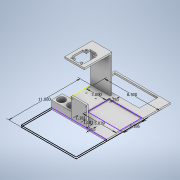
# Autodesk Inventor part: liquid cell loader tray thing
Saved by Autodesk Inventor 2020 (Build 240168000, 168)
## iProperties
Created: 2021-12-08
Part Number: liquid cell loader tray thing
Material: Generic
Document SubType Name: Modeling
Designer: pab2
Density: 1 g/cm^3
Appearance: Default
Author: pab2
Autodesk Inventor part; units mm, degrees
ref_plane "YZ Plane" through (0, 0, 0) normal (1, 0, 0) x (0, 1, 0)
ref_plane "XZ Plane" through (0, 0, 0) normal (0, 1, 0) x (-1, 0, 0)
ref_plane "XY Plane" through (0, 0, 0) normal (0, 0, 1) x (1, 0, 0)
sketch "Sketch1" plane through (0, 0, 0) normal (0, 1, 0) x (-1, 0, 0)
  line L0 (0, 0) -> (215.9, 0)
  line L1 (215.9, 0) -> (215.9, -279.4)
  line L2 (215.9, -279.4) -> (0, -279.4)
  line L3 (0, -279.4) -> (0, 0)
  line L4 (215.9, -279.4) -> (139.7, -279.4)
  line L5 (139.7, -279.4) -> (139.7, -273.05)
  line L6 (139.7, -273.05) -> (215.9, -273.05)
  line L7 (215.9, -273.05) -> (215.9, -279.4)
  dimension "d0" = 215.9
  dimension "d1" = 279.4
  dimension "d2" = 76.2
  dimension "d3" = 6.35
  constraints: 16 end point, 4 parallel, 2 horizontal, 2 perpendicular
  measures "d0" distance of L1.end L2.end
  measures "d1" distance of L0.end L1.end
  measures "d2" distance of L5.end L6.end
  measures "d3" distance of L4.end L5.end
extrude "Extrusion1" add sketch "Sketch1" along normal blind 152.4 contours L1 L2 L5 L6
extrude "Extrusion2" add sketch "Sketch1" along normal blind 6.35 contours L0 L1 L6 L5 L2 L3
sketch "Sketch2" plane through (-215.9, 152.4, -273.05) normal (0, 0, 1) x (1, 0, 0)
  line L0 (76.2, 0) -> (0, 0) projected
  line L1 (76.2, -146.05) -> (76.2, 0) projected
  line L2 (0, 0) -> (76.2, 0)
  line L3 (76.2, 0) -> (76.2, -6.35)
  line L4 (76.2, -6.35) -> (0, -6.35)
  line L5 (0, -6.35) -> (0, 0)
  point P0 (215.9, -152.4)
  dimension "d8" = 6.35
  constraints: 8 end point, 2 parallel, 1 horizontal, 1 perpendicular, 1 point on line
  measures "d8" distance of L2.end L3.end
extrude "Extrusion3" add sketch "Sketch2" along normal blind 101.6
sketch "Sketch3" plane through (0, 152.4, 0) normal (0, 1, 0) x (1, 0, 0)
  line L0 (-215.9, 273.05) -> (-215.9, 0) projected
  line L1 (-139.7, 171.45) -> (-215.9, 171.45)
  line L2 (-215.9, 171.45) -> (-215.9, 180.975)
  line L3 (-215.9, 180.975) -> (-139.7, 180.975)
  line L4 (-139.7, 180.975) -> (-139.7, 171.45)
  line L5 (-177.8, 180.975) -> (-196.088, 180.975)
  line L6 (-177.8, 180.975) -> (-159.512, 180.975)
  line L7 (-159.512, 180.975) -> (-159.512, 236.601)
  line L8 (-196.088, 180.975) -> (-196.088, 236.601)
  point P0 (0, 0)
  dimension "d11" = 9.525
  dimension "d12" = 18.288
  dimension "d13" = 18.288
  dimension "d14" = 55.626
  dimension "d15" = 55.626
  constraints: 16 end point, 3 point on line, 2 parallel, 2 perpendicular, 1 horizontal, 1 midpoint, 1 vertical
  measures "d11" distance of L1.end L2.end
  measures "d12" distance of L5.start L5.end
  measures "d13" distance of L5.start L6.end
  measures "d14" distance of L6.end L7.end
  measures "d15" distance of L5.end L8.end
hole "Hole1" at (-196.088, 152.4, -236.601) at (-159.512, 152.4, -236.601) at (-159.512, 152.4, -180.975) at (-196.088, 152.4, -180.975) direction (0, -1, 0) diameter 4.4958 depth 146.05 tip angle 118 start extended yes counterbore diameter 7.9502 counterbore depth 4.1656 clearance for "Socket Head Cap Screw" size "#8" standard "Ansi Unified Screw Threads"
sketch "Sketch4" plane through (0, 152.4, 0) normal (0, 1, 0) x (1, 0, 0)
  line L0 (-215.9, 279.4) -> (-215.9, 171.45) projected
  line L1 (-215.9, 171.45) -> (-215.9, 187.325)
  line L2 (-215.9, 187.325) -> (-203.2, 187.325)
  line L3 (-203.2, 187.325) -> (-153.924, 187.325)
  line L4 (-153.924, 187.325) -> (-153.924, 229.8268)
  line L5 (-153.924, 229.8268) -> (-203.2, 229.8268)
  line L6 (-203.2, 229.8268) -> (-203.2, 187.325)
  line L7 (-190.2248, 177.0242) -> (-165.5159, 177.0242)
  line L8 (-165.5159, 177.0242) -> (-165.5159, 245.3968)
  line L9 (-165.5159, 245.3968) -> (-190.2248, 245.3968)
  line L10 (-190.2248, 245.3968) -> (-190.2248, 177.0242)
  point P0 (0, 0)
  point P1 (-165.5159, 187.325)
  point P2 (-165.5159, 229.8268)
  point P3 (-190.2248, 229.8268)
  point P4 (-190.2248, 187.325)
  dimension "d23" = 15.875
  dimension "d24" = 12.7
  dimension "d25" = 49.276
  constraints: 20 end point, 4 parallel, 3 perpendicular, 2 horizontal, 1 point on line
  measures "d23" distance of L0.end L1.end
  measures "d24" distance of L1.end L2.end
  measures "d25" distance of L5.end L4.end
extrude "Extrusion4" cut sketch "Sketch4" against normal blind 101.6
sketch "Sketch5" plane through (0, 6.35, 0) normal (0, 1, 0) x (1, 0, 0)
  line L0 (-132.2495, 261.4471) -> (-4.2495, 261.4471)
  line L1 (-4.2495, 261.4471) -> (-4.2495, 175.4471)
  line L2 (-4.2495, 175.4471) -> (-132.2495, 175.4471)
  line L3 (-132.2495, 175.4471) -> (-132.2495, 261.4471)
  line L4 (-215.9, 273.05) -> (-215.9, 0) projected
  line L5 (-215.9, 161.7513) -> (-138.3533, 161.7513)
  line L6 (-138.3533, 161.7513) -> (-138.3533, 119.3637)
  line L7 (-138.3533, 119.3637) -> (-215.9, 119.3637)
  line L8 (-215.9, 119.3637) -> (-215.9, 161.7513)
  line L9 (-215.9, 119.3637) -> (0, 119.3637)
  line L10 (0, 119.3637) -> (0, 0)
  line L11 (0, 0) -> (-215.9, 0)
  line L12 (-215.9, 0) -> (-215.9, 119.3637)
  line L13 (-107.95, 119.3637) -> (-77.95, 119.3637)
  line L14 (-77.95, 119.3637) -> (-77.95, 125.7137)
  line L15 (-77.95, 125.7137) -> (-107.95, 125.7137)
  line L16 (-107.95, 125.7137) -> (-107.95, 119.3637)
  line L17 (-107.95, 119.3637) -> (-137.95, 119.3637)
  line L18 (-137.95, 119.3637) -> (-137.95, 125.7137)
  line L19 (-137.95, 125.7137) -> (-107.95, 125.7137)
  line L20 (-107.95, 125.7137) -> (-107.95, 119.3637)
  dimension "d28" = 128
  dimension "d29" = 86
  dimension "d42" = 30
  dimension "d43" = 6.35
  dimension "d44" = 30
  constraints: 40 end point, 10 parallel, 5 horizontal, 5 perpendicular, 1 midpoint, 1 point on line
  measures "d28" distance of L1.end L2.end
  measures "d29" distance of L0.end L1.end
  measures "d42" distance of L15.end L14.end
  measures "d43" distance of L14.end L13.end
  measures "d44" distance of L18.end L19.end
extrude "Extrusion5" cut sketch "Sketch5" against normal blind 3.81 contours L0 L1 L2 L3
extrude "Extrusion6" add sketch "Sketch5" along normal blind 25.4 contours L5 L6 L7 L4
sketch "Sketch6" plane through (0, 31.75, 0) normal (0, 1, 0) x (1, 0, 0)
  line L0 (-138.3533, 161.7513) -> (-138.3533, 119.3637) projected
  line L1 (-138.3533, 140.5575) -> (-157.4033, 140.5575)
  line L2 (-215.9, 279.4) -> (-215.9, 0) projected
  line L3 (-138.3533, 140.5575) -> (-119.3033, 140.5575) construction
  circle A0 centre (-157.4033, 140.5575) radius 14.5
  line L4 (-215.9, 139.7) -> (-196.85, 139.7)
  line L5 (-215.9, 139.7) -> (-196.85, 139.7) construction
  circle A1 centre (-196.85, 139.7) radius 14.5
  point P0 (0, 0)
  dimension "d34" = 19.05
  dimension "d35" = 180
  dimension "d36" = 29
  dimension "d37" = 19.05
  dimension "d38" = 0
  dimension "d39" = 29
  constraints: 8 end point, 3 horizontal, 2 centre point, 2 coincident, 2 collinear, 2 midpoint, 1 perpendicular
  measures "d34" distance of L1.start L1.end
  measures "d35" angle of L1 L3
  measures "d36" diameter of A0
  measures "d37" distance of L4.start L4.end
  measures "d38" distance between parallel lines of L4 L5
  measures "d39" diameter of A1
extrude "Extrusion7" cut sketch "Sketch6" against normal blind 29.21
extrude "Extrusion8" add sketch "Sketch5" along normal blind 76.2 contours L18 L19 L16 L9 | L16 L15 L14 L9
extrude "Extrusion9" cut sketch "Sketch5" against normal blind 76.2 contours L7 L9 L10 L11 L4
sketch "Sketch7" plane through (-215.9, 0, -119.3637) normal (0, 0, 1) x (1, 0, 0)
  line L0 (77.95, 82.55) -> (137.95, 82.55) projected
  line L1 (107.95, 82.55) -> (134.45, 82.55)
  line L2 (134.45, 82.55) -> (134.45, 76.2)
  line L3 (134.45, 76.2) -> (107.95, 76.2)
  line L4 (107.95, 76.2) -> (107.95, 82.55)
  line L5 (107.95, 82.55) -> (81.45, 82.55)
  line L6 (81.45, 82.55) -> (81.45, 76.2)
  line L7 (81.45, 76.2) -> (107.95, 76.2)
  line L8 (107.95, 76.2) -> (107.95, 82.55)
  point P0 (215.9, 0)
  point P1 (113.2316, 50.6759)
  point P2 (91.9547, 40.3217)
  dimension "d49" = 26.5
  dimension "d50" = 6.35
  dimension "d51" = 26.5
  constraints: 16 end point, 4 parallel, 2 horizontal, 2 perpendicular, 1 midpoint
  measures "d49" distance of L2.end L3.end
  measures "d50" distance of L1.end L2.end
  measures "d51" distance of L7.end L6.end
hole "Hole2" at (-134.45, 76.2, -119.3637) at (-81.45, 76.2, -119.3637) direction (0, 0, -1) diameter 3.683 depth 6.35 tip angle 118 start extended yes thread size "10-24 UNC" class "2B" standard "ANSI Unified Screw Threads"
sketch "Sketch9" plane through (-139.7, 152.4, -279.4) normal (0, 0, -1) x (-1, 0, 0)
  line L0 (-139.7, -146.05) -> (0, -146.05) projected
  line L1 (-139.7, -146.05) -> (76.2457, -146.05)
  line L2 (76.2457, -146.05) -> (76.2457, -152.4)
  line L3 (76.2457, -152.4) -> (-139.7, -152.4)
  line L4 (-139.7, -152.4) -> (-139.7, -146.05)
  constraints: 8 end point, 2 parallel, 1 horizontal, 1 perpendicular
extrude "Extrusion10" add sketch "Sketch9" along normal blind 88.9
sketch "Sketch10" plane through (0, 6.35, 0) normal (0, 1, 0) x (1, 0, 0)
  line L0 (-215.9457, 368.3) -> (0, 368.3) projected
  line L1 (-215.9457, 368.3) -> (-215.9457, 361.95)
  line L2 (-215.9457, 279.4) -> (-215.9457, 368.3) projected
  line L3 (-215.9457, 361.95) -> (-209.5957, 361.95)
  line L4 (-209.5957, 361.95) -> (-41.3207, 361.95)
  line L5 (-41.3207, 361.95) -> (-41.3207, 288.925)
  line L6 (-41.3207, 288.925) -> (-209.5957, 288.925)
  line L7 (-209.5957, 288.925) -> (-209.5957, 361.95)
  point P0 (0, 0)
  dimension "d61" = 6.35
  dimension "d62" = 6.35
  dimension "d63" = 168.275
  dimension "d64" = 73.025
  constraints: 12 end point, 2 parallel, 2 perpendicular, 1 horizontal, 1 point on line
  measures "d61" distance of L0.start L1.end
  measures "d62" distance of L1.end L3.end
  measures "d63" distance of L5.end L6.end
  measures "d64" distance of L4.end L5.end
extrude "Extrusion11" cut sketch "Sketch10" against normal blind 6.35
body "Solid1"
